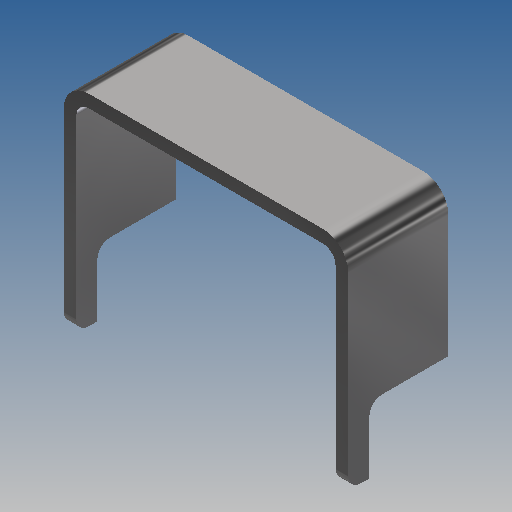
# Autodesk Inventor part: DD_KVD_002_05
Saved by Autodesk Inventor 2017.3 (Build 213256000, 256)
## iProperties
Created: 2023-11-02
Part Number: DD_KVD_002_05
Material: Nerezová ocel
Document SubType Name: Sheet Metal
Designer: Darena
Density: 8 g/cm^3
Sheet Metal Rule: Výchozí_mm
Appearance: Pololeštěná
Flat Pattern Width: 4.75 cm
Flat Pattern Length: 31.7143 cm
Flat Pattern Area: 150.643 cm^2
Sheet Metal Width: 47,500 mm
Sheet Metal Length: 317,143 mm
Sheet Metal Area: 15064,310 mm^2
Author: Darena
Autodesk Inventor part; units mm, degrees
ref_plane "YZ Plane" through (0, 0, 0) normal (1, 0, 0) x (0, 1, 0)
ref_plane "XZ Plane" through (0, 0, 0) normal (0, 1, 0) x (-1, 0, 0)
ref_plane "XY Plane" through (0, 0, 0) normal (0, 0, 1) x (1, 0, 0)
sketch "Náčrt2" plane through (0, 0, 0) normal (0, 1, 0) x (-1, 0, 0)
  line L0 (67.5, 23.75) -> (-67.5, 23.75)
  line L1 (-67.5, 23.75) -> (-67.5, -23.75)
  line L2 (-67.5, -23.75) -> (67.5, -23.75)
  line L3 (67.5, -23.75) -> (67.5, 23.75)
  point P0 (0, 0)
  point P1 (67.5, 0)
  point P2 (0, 23.75)
  dimension "d0" = 135
  dimension "d1" = 47.5
  constraints: 8 end point, 2 midpoint, 2 parallel, 1 horizontal, 1 horizontal alignment, 1 perpendicular, 1 vertical alignment
  measures "d0" distance of L0.start L0.end
  measures "d1" distance of L2.end L0.start
extrude "Vysunutí1" add sketch "Náčrt2" along normal blind 6
sketch "Náčrt3" plane through (61.5, 6, 23.75) normal (1, 0, 0) x (0, 1, 0)
  line L0 (0, -47.5) -> (0, 0)
  line L1 (0, 0) -> (-70, 0)
  line L2 (-70, 0) -> (-70, -47.5)
  line L3 (-70, -47.5) -> (0, -47.5)
  constraints: 6 end point, 1 horizontal, 1 perpendicular, 1 vertical
edge flange "Obruba1" height 70 angle 90 thickness 6 bend radius 6 thickness toward (1, 0, 0) relief tear relief width 6 relief depth 3 corner gap 6 corner form 0 edges at (67.5, 0, 0) (-67.5, 0, 0) wall of the first edge with corners at (61.5, 6, -23.75) (61.5, 6, 23.75) (61.5, -64, 23.75) (61.5, -64, -23.75)
bend "Ohyb1"
corner "Roh1"
sketch "Náčrt4" plane through (-67.5, -64, -23.75) normal (0, -1, 0) x (1, 0, 0)
  line L0 (0, 47.5) -> (0, 0) construction
  line L1 (6, 0) -> (0, 0) construction
  line L2 (6, 47.5) -> (6, 0) construction
  line L3 (6, 47.5) -> (0, 47.5) construction
  line L4 (135, 0) -> (135, 47.5) construction
  line L5 (129, 47.5) -> (135, 47.5) construction
  line L6 (129, 0) -> (129, 47.5) construction
  line L7 (129, 0) -> (135, 0) construction
  line L8 (0, 47.5) -> (0, 0) projected
  line L9 (0, 47.5) -> (6, 47.5)
  line L10 (6, 47.5) -> (6, 37.5)
  line L11 (6, 37.5) -> (0, 37.5)
  line L12 (0, 37.5) -> (0, 47.5)
  line L13 (135, 47.5) -> (129, 47.5)
  line L14 (129, 47.5) -> (129, 37.5)
  line L15 (129, 37.5) -> (135, 37.5)
  line L16 (135, 37.5) -> (135, 47.5)
  point P0 (67.5, 23.75)
  dimension "d18" = 10
  constraints: 16 end point, 4 parallel, 2 horizontal, 2 perpendicular, 2 point on line, 1 collinear
  measures "d18" distance between parallel lines of L11 L3
extrude "Vysunutí2" add sketch "Náčrt4" along normal blind 31.5
fillet "Zaoblení2" radius 6 4 edges at (64.5, -64, 13.75) (-64.5, -64, 13.75) (-64.5, -95.5, 23.75) (64.5, -95.5, 23.75)
equation "\"d4\" = ŠířkaVýštipu"
equation "\"d5\" = HloubkaVýštipu"
equation "\"d6\" = MinimálníZbytek"
equation "\"d7\" = PoloměrOhybu"
equation "\"d10\" = PoloměrOhybu"
equation "\"d11\" = VelikostRohovéhoVýštipu"
equation "\"d12\" = VelikostMezery"
equation "\"d13\" = VelikostJacobihoPoloměru"
equation "\"PoloměrOhybu\" = Tloušťka"
equation "\"ŠířkaVýštipu\" = Tloušťka"
equation "\"HloubkaVýštipu\" = 0.5 * Tloušťka"
equation "\"VelikostRohovéhoVýštipu\" = 4 * Tloušťka"
equation "\"MinimálníZbytek\" = 2 * Tloušťka"
equation "\"PřechodovýPoloměr\" = PoloměrOhybu"
equation "\"VelikostJacobihoPoloměru\" = PoloměrOhybu"
equation "\"VelikostMezery\" = Tloušťka"
equation "\"Tloušťka\" = 6"
